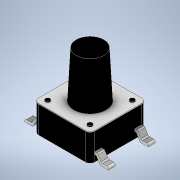
# Autodesk Inventor part: TactSwitch_6x6_8mm_SMD
Saved by Autodesk Inventor 2021 (Build 250183000, 183)
## iProperties
Created: 2021-07-21
Part Number: TactSwitch_6x6_8mm_SMD
Material: Generic
Document SubType Name: Modeling
Designer: ermoz
Density: 1 g/cm^3
Appearance: Default
Author: ermoz
Autodesk Inventor part; units mm, degrees
note: some values were not read from the file. Chosen so that the rebuilt part matches the saved one: second side of "Extrusion4".
ref_plane "YZ Plane" through (0, 0, 0) normal (1, 0, 0) x (0, 1, 0)
ref_plane "XZ Plane" through (0, 0, 0) normal (0, 1, 0) x (-1, 0, 0)
sketch "Sketch1" plane through (0, 0, 0) normal (0, 1, 0) x (-1, 0, 0)
  line L0 (-3.05, 3.05) -> (3.05, 3.05)
  line L1 (3.05, 3.05) -> (3.05, -3.05)
  line L2 (3.05, -3.05) -> (-3.05, -3.05)
  line L3 (-3.05, -3.05) -> (-3.05, 3.05)
  line L4 (-3.05, 3.05) -> (3.05, -3.05) construction
  line L5 (3.05, 3.05) -> (-3.05, -3.05) construction
  point P0 (0, 0)
  dimension "d0" = 6.1
  constraints: 12 end point, 2 midpoint, 2 parallel, 2 perpendicular, 1 horizontal
  measures "d0" distance of L1.end L2.end
extrude "Extrusion1" add sketch "Sketch1" along normal blind 2.9
fillet "Fillet1" radius 0.5 4 edges at (3.05, 1.45, 3.05) (3.05, 1.45, -3.05) (-3.05, 1.45, 3.05) (-3.05, 1.45, -3.05)
sketch "Sketch2" plane through (0, 2.9, 0) normal (0, 1, 0) x (1, 0, 0)
  arc A0 (-2.55, 3.05) -> (-3.05, 2.55) centre (-2.55, 2.55) ccw projected
  line L0 (-3.05, 2.55) -> (-3.05, -2.55) projected
  arc A1 (-3.05, -2.55) -> (-2.55, -3.05) centre (-2.55, -2.55) ccw projected
  line L1 (-2.55, -3.05) -> (2.55, -3.05) projected
  arc A2 (2.55, -3.05) -> (3.05, -2.55) centre (2.55, -2.55) ccw projected
  line L2 (3.05, -2.55) -> (3.05, 2.55) projected
  arc A3 (3.05, 2.55) -> (2.55, 3.05) centre (2.55, 2.55) ccw projected
  line L3 (2.55, 3.05) -> (-2.55, 3.05) projected
  circle A4 centre (-2.3, -2.3) radius 0.25
  line L4 (0, 0) -> (0, -0.8572)
  line L5 (0, 0) -> (0.9722, 0)
  circle A5 centre (-2.3, 2.3) radius 0.25
  circle A6 centre (2.3, -2.3) radius 0.25
  circle A7 centre (2.3, 2.3) radius 0.25
  circle A8 centre (0, 0) radius 1.75
  dimension "d5" = 0.75
  dimension "d6" = 0.75
  dimension "d11" = 3.5
  constraints: 7 symmetric about line, 5 centre point, 4 end point, 1 coincident, 1 horizontal, 1 vertical, 3 other
  measures "d5" distance from line of L1 A4.centre
  measures "d6" distance from line of L0 A4.centre
  measures "d11" diameter of A8
extrude "Extrusion2" add sketch "Sketch2" along normal blind 0.2 contours A4 | A5 | A6 | A7
extrude "Extrusion3" add sketch "Sketch2" along normal blind 0.1 separate body
ref_plane "Work Plane1" through (0, 3, 3.05) normal (1, 0, 0) x (0, 1, 0)
sketch "Sketch3" plane through (0, 3, 3.05) normal (1, 0, 0) x (0, 1, 0)
  line L0 (-0.1, -0.5) -> (-0.1, -5.6) projected
  line L1 (-0.1, -3.05) -> (5, -3.05)
  line L2 (5, -3.05) -> (5, -4.55)
  line L3 (5, -4.55) -> (-0.1, -4.8)
  line L4 (0, -4.8) -> (-0.1, -4.8) projected
  line L5 (-0.1, -4.8) -> (-0.1, -3.05)
  line L6 (-3, -0.5) -> (-3, -5.6) projected
  point P0 (-3, -3.05)
  point P1 (-0.1, -4.8)
  dimension "d12" = 1.5
  dimension "d13" = 8
  constraints: 8 end point, 1 horizontal, 1 midpoint, 1 parallel, 1 perpendicular, 1 point on line
  measures "d12" distance of L1.end L2.end
  measures "d13" distance between parallel lines of L6 L2
revolve "Revolution1" add sketch "Sketch3" angle 360 about axis through (0, 2.9, 0) along (0, 1, 0) separate body
sketch "Sketch4" plane through (0, 0, 0) normal (0, -1, 0) x (1, 0, 0)
  line L0 (-3.05, -2.55) -> (-3.05, 2.55) projected
  line L1 (-3.05, 2.55) -> (-4.55, 2.55)
  line L2 (-4.55, 2.55) -> (-4.55, 1.8)
  line L3 (-4.55, 1.8) -> (-3.05, 1.8)
  line L4 (-3.05, 1.8) -> (-3.05, 2.55)
  line L5 (-2.55, 3.05) -> (2.55, 3.05) projected
  line L6 (0, 0) -> (-0.9162, 0)
  line L7 (0, 0) -> (0, 1.1643)
  line L8 (-3.05, -2.55) -> (-4.55, -2.55)
  line L9 (-4.55, -2.55) -> (-4.55, -1.8)
  line L10 (-4.55, -1.8) -> (-3.05, -1.8)
  line L11 (-3.05, -1.8) -> (-3.05, -2.55)
  line L12 (3.05, -2.55) -> (3.05, 2.55)
  line L13 (3.05, 2.55) -> (4.55, 2.55)
  line L14 (4.55, 2.55) -> (4.55, 1.8)
  line L15 (4.55, 1.8) -> (3.05, 1.8)
  line L16 (3.05, 1.8) -> (3.05, 2.55)
  line L17 (3.05, -2.55) -> (4.55, -2.55)
  line L18 (4.55, -2.55) -> (4.55, -1.8)
  line L19 (4.55, -1.8) -> (3.05, -1.8)
  line L20 (3.05, -1.8) -> (3.05, -2.55)
  dimension "d15" = 1.5
  dimension "d16" = 0.75
  dimension "d17" = 0.5
  constraints: 38 end point, 16 symmetric about line, 2 horizontal, 2 parallel, 2 point on line, 1 perpendicular, 1 vertical
  measures "d15" distance of L3.end L2.end
  measures "d16" distance of L2.end L1.end
  measures "d17" distance between parallel lines of L5 L1
extrude "Extrusion4" add sketch "Sketch4" against normal blind 1 separate body
sketch "Sketch5" plane through (-4.55, 0, 2.55) normal (0, 0, 1) x (1, 0, 0)
  line L0 (0, 0) -> (0.8968, 0)
  line L1 (0.8968, 0) -> (1.1421, 0.4226)
  line L2 (1.5, 1) -> (1.1638, 1)
  line L3 (1.1638, 1) -> (0.7514, 0.2896)
  line L4 (0.7514, 0.2896) -> (0, 0.289)
  line L5 (0, 0.289) -> (0, 0)
  line L6 (1.1421, 0.4226) -> (1.3095, 0.711)
  line L7 (1.3095, 0.711) -> (1.5, 0.711)
  line L8 (1.5, 1) -> (1.5, 0.711)
  line L9 (4.55, 0) -> (4.55, -1.1807)
  line L10 (0, 1) -> (1.5, 1) projected
  line L11 (1.1638, 1) -> (0, 1)
  line L12 (0, 1) -> (0, 1)
  line L13 (0, 0.289) -> (0, 1)
  line L14 (1.5, 0) -> (0, 0) projected
  line L15 (0.8968, 0) -> (1.5, 0)
  line L16 (1.5, 0) -> (1.5, 0)
  line L17 (1.5, 0) -> (1.5, 2.9) projected
  line L18 (1.5, 0.711) -> (1.5, 0)
  line L19 (9.1, 0) -> (8.2032, 0)
  line L20 (8.2032, 0) -> (7.9579, 0.4226)
  line L21 (7.6, 1) -> (7.9362, 1)
  line L22 (7.9362, 1) -> (8.3486, 0.2896)
  line L23 (8.3486, 0.2896) -> (9.1, 0.289)
  line L24 (9.1, 0.289) -> (9.1, 0)
  line L25 (7.9579, 0.4226) -> (7.7905, 0.711)
  line L26 (7.7905, 0.711) -> (7.6, 0.711)
  line L27 (7.6, 1) -> (7.6, 0.711)
  line L28 (9.1, 1) -> (7.6, 1)
  line L29 (7.9362, 1) -> (9.1, 1)
  line L30 (9.1, 1) -> (9.1, 1)
  line L31 (9.1, 0.289) -> (9.1, 1)
  line L32 (7.6, 0) -> (9.1, 0)
  line L33 (8.2032, 0) -> (7.6, 0)
  line L34 (7.6, 0) -> (7.6, 0)
  line L35 (7.6, 0.711) -> (7.6, 0)
  point P0 (1.1638, 1)
  constraints: 66 end point, 11 symmetric about line, 4 collinear, 2 parallel, 2 perpendicular, 1 vertical
extrude "Extrusion5" cut sketch "Sketch5" against normal through all contours L1 L6 L7 L17 L14 | L13 L10 L3 L4 | L32 L35 L26 L25 L20 | L23 L22 L28 L31 bodies 4
fillet "Fillet2" radius 0.2 20 edges at (-3.3862, 1, -2.175) (-3.7986, 0.2896, -2.175) (-4.55, 0.289, -2.175) (-3.6532, 0, -2.175) (-3.2405, 0.711, -2.175) (-3.2405, 0.711, 2.175) (-3.6532, 0, 2.175) (-3.3862, 1, 2.175) (-3.7986, 0.2896, 2.175) (-4.55, 0.289, 2.175) (3.3862, 1, 2.175) (3.7986, 0.2896, 2.175) (3.2405, 0.711, 2.175) (3.6532, 0, 2.175) (4.55, 0.289, 2.175) (4.55, 0.289, -2.175) (3.7986, 0.2896, -2.175) (3.3862, 1, -2.175) (3.6532, 0, -2.175) (3.2405, 0.711, -2.175)
body "Solid1"
body "Solid2"
body "Solid3"
body "Solid4"
